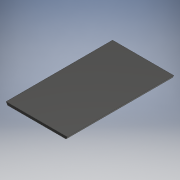
# Autodesk Inventor part: BA11
Saved by Autodesk Inventor 2017 (Build 210142000, 142)
## iProperties
Created: 2019-05-29
Part Number: BA11
Material: Wood (Cherry)
Document SubType Name: Modeling
Designer: Dell
Density: 0.63 g/cm^3
Appearance: Smooth - Black
Author: Dell
Autodesk Inventor part; units mm, degrees
ref_plane "YZ Plane" through (0, 0, 0) normal (1, 0, 0) x (0, 1, 0)
ref_plane "XZ Plane" through (0, 0, 0) normal (0, 1, 0) x (-1, 0, 0)
ref_plane "XY Plane" through (0, 0, 0) normal (0, 0, 1) x (1, 0, 0)
sketch "Sketch1" plane through (0, 0, 0) normal (0, 0, 1) x (1, 0, 0)
  line L0 (0, 0) -> (310.8917, 0)
  line L1 (310.8917, 0) -> (310.8917, 539.75)
  line L2 (310.8917, 539.75) -> (0, 539.75)
  line L3 (0, 539.75) -> (0, 0)
  dimension "d0" = 539.75
  dimension "d1" = 310.8917
  constraints: 8 end point, 2 parallel, 1 horizontal, 1 perpendicular
  measures "d0" distance of L1.end L0.end
  measures "d1" distance of L1.end L2.end
extrude "Extrusion1" add sketch "Sketch1" along normal blind 12.7
sketch "Sketch2" plane through (0, 539.75, 0) normal (0, 1, 0) x (1, 0, 0)
  line L0 (0, -12.7) -> (310.8917, -12.7) projected
  line L1 (0, -12.7) -> (7.3323, 0)
  line L2 (0, 0) -> (310.8917, 0) projected
  line L3 (0, 0) -> (7.3323, 0)
  line L4 (0, 0) -> (0, -12.7)
  line L5 (310.8917, -12.7) -> (303.5593, 0)
  line L6 (310.8917, 0) -> (303.5593, 0)
  line L7 (310.8917, 0) -> (310.8917, -12.7) projected
  line L8 (310.8917, 0) -> (310.8917, -12.7)
  dimension "d4" = 30
  dimension "d5" = 30
  constraints: 12 end point, 2 collinear, 2 point on line, 1 perpendicular, 1 vertical
  measures "d4" angle of L4 L1
  measures "d5" angle of L5 L7
extrude "Extrusion2" cut sketch "Sketch2" against normal through all contours L4 L2 L1 | L5 L2 L7
body "Solid1"
